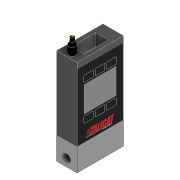
# Autodesk Inventor part: alicat_presion
Saved by Autodesk Inventor 2022 (Build 260153000, 153)
## iProperties
Created: 2022-11-14
Part Number: alicat_presion
Material: Generic
Document SubType Name: Modeling
Designer: ferna
Density: 1 g/cm^3
Appearance: Default
Author: ferna
Autodesk Inventor part; units mm, degrees
ref_plane "YZ Plane" through (0, 0, 0) normal (1, 0, 0) x (0, 1, 0)
ref_plane "XZ Plane" through (0, 0, 0) normal (0, 1, 0) x (-1, 0, 0)
ref_plane "XY Plane" through (0, 0, 0) normal (0, 0, 1) x (1, 0, 0)
sketch "Sketch1" plane through (0, 0, 0) normal (0, 1, 0) x (-1, 0, 0)
  line L0 (0, 0) -> (27, 0)
  line L1 (27, 0) -> (27, -61)
  line L2 (27, -61) -> (0, -61)
  line L3 (0, -61) -> (0, 0)
  dimension "d0" = 27
  dimension "d1" = 61
  constraints: 8 end point, 2 parallel, 1 horizontal, 1 perpendicular
  measures "d0" distance of L1.end L2.end
  measures "d1" distance of L0.end L1.end
extrude "Extrusion1" add sketch "Sketch1" along normal blind 125
sketch "Sketch2" plane through (0, 0, 0) normal (1, 0, 0) x (0, 0, -1)
  line L0 (61, 0) -> (0, 0) projected
  line L1 (61, 0) -> (61, 125) projected
  line L2 (0, 0) -> (61, 0)
  line L3 (61, 0) -> (61, 30)
  line L4 (61, 30) -> (0, 30)
  line L5 (0, 30) -> (0, 0)
  dimension "d4" = 30
  constraints: 8 end point, 2 parallel, 1 horizontal, 1 perpendicular, 1 point on line
  measures "d4" distance of L3.end L2.end
split body "Split1" sketch "Sketch2" result two bodies curves L4 L5 L2 L3 first body at (-0.5, 10, -20.3333)
sketch "Sketch3" plane through (0, 0, 0) normal (0, -1, 0) x (1, 0, 0)
  line L0 (-27, 0) -> (0, 0) projected
  line L1 (-27, -61) -> (-27, 0) projected
  line L2 (0, 0) -> (-27, -61)
  line L3 (-27, -61) -> (-22.9525, -51.8557)
  line L4 (0, 0) -> (-4.0475, -9.1443)
  circle A0 centre (-4.0475, -9.1443) radius 2
  circle A1 centre (-22.9525, -51.8557) radius 2
  line L5 (0, -61) -> (-27, -61) projected
  line L6 (-27, 0) -> (0, -61)
  line L7 (0, -61) -> (-3.238, -53.6846)
  line L8 (-27, 0) -> (-23.762, -7.3154)
  circle A2 centre (-23.762, -7.3154) radius 2
  circle A3 centre (-3.238, -53.6846) radius 2
  dimension "d5" = 10
  dimension "d6" = 10
  dimension "d7" = 4
  dimension "d8" = 4
  dimension "d14" = 8
  dimension "d15" = 8
  dimension "d16" = 4
  constraints: 12 end point, 4 centre point, 4 coincident, 4 point on line
  measures "d5" distance of L1.start L3.end
  measures "d6" distance of L0.end L4.end
  measures "d7" diameter of A0
  measures "d8" diameter of A1
  measures "d14" distance of L5.start L7.end
  measures "d15" distance of L0.start L8.end
  measures "d16" diameter of A3
extrude "Extrusion2" cut sketch "Sketch3" against normal blind 10 contours A2 L6 | L6 A2 | A3 L6 | L6 A3 bodies 2
sketch "Sketch4" plane through (-27, 0, 0) normal (0, 0, 1) x (1, 0, 0)
  line L0 (0, 0) -> (0, 30) projected
  line L1 (0, 0) -> (13.5, 0)
  line L2 (0, 0) -> (27, 0) projected
  line L3 (13.5, 0) -> (13.5, 10)
  circle A0 centre (13.5, 10) radius 5
  dimension "d11" = 10
  constraints: 4 end point, 1 centre point, 1 coincident, 1 midpoint, 1 perpendicular
  measures "d11" distance of L1.end L3.end
extrude "Extrusion3" cut sketch "Sketch4" against normal blind 10 bodies 2
sketch "Sketch12" plane through (0, 125, 0) normal (1, 0, 0) x (0, 0, -1)
  line L0 (0.5745, -8.0578) -> (59.8412, -8.0578) construction
  line L1 (59.8412, -8.0578) -> (59.8412, -95.0528) construction
  line L2 (59.8412, -95.0528) -> (0.5745, -95.0528) construction
  line L3 (0.5745, -95.0528) -> (0.5745, -8.0578) construction
  point P0 (0, -125)
  constraints: 2 other
decal "Decal2"
sketch "Sketch13" plane through (0, 125, 0) normal (0, 1, 0) x (1, 0, 0)
  line L0 (-27, 0) -> (0, 0) projected
  line L1 (0, 0) -> (-13.5, 0)
  line L2 (-13.5, 0) -> (-13.5, 30.5)
  line L3 (0, 61) -> (-27, 61) projected
  line L4 (-21.825, 46.4) -> (-5.175, 46.4)
  line L5 (-5.175, 46.4) -> (-5.175, 14.6)
  line L6 (-5.175, 14.6) -> (-21.825, 14.6)
  line L7 (-21.825, 14.6) -> (-21.825, 46.4)
  line L8 (-21.825, 46.4) -> (-5.175, 14.6) construction
  line L9 (-5.175, 46.4) -> (-21.825, 14.6) construction
  dimension "d39" = 30.5
  dimension "d40" = 16.65
  dimension "d41" = 31.8
  constraints: 16 end point, 3 midpoint, 2 parallel, 2 perpendicular, 1 horizontal
  measures "d39" distance of L1.end L2.end
  measures "d40" distance of L5.end L6.end
  measures "d41" distance of L4.end L5.end
extrude "Extrusion4" cut sketch "Sketch13" against normal blind 16.2 bodies 3
sketch "Sketch14" plane through (0, 125, 0) normal (0, 1, 0) x (1, 0, 0)
  line L0 (-5.175, 14.6) -> (-21.825, 14.6) projected
  line L1 (-13.5, 14.6) -> (-13.5, 7.3)
  line L2 (-27, 0) -> (0, 0) projected
  circle A0 centre (-13.5, 7.3) radius 4
  dimension "d44" = 7.3
  dimension "d45" = 8
  constraints: 2 end point, 1 centre point, 1 coincident, 1 midpoint, 1 perpendicular
  measures "d44" distance of L1.start L1.end
  measures "d45" diameter of A0
extrude "Extrusion5" cut sketch "Sketch14" against normal blind 1 bodies 3
sketch "Sketch15" plane through (-13.5, 124, -7.3) normal (0, 1, 0) x (1, 0, 0)
  circle A0 centre (0, 0) radius 3
  point P0 (13.5, -7.3)
  dimension "d48" = 6
  constraints: 1 centre point
  measures "d48" diameter of A0
extrude "Extrusion6" cut sketch "Sketch15" against normal blind 7 bodies 3
sketch "Sketch16" plane through (0, 125, 0) normal (0, 1, 0) x (1, 0, 0)
  circle A0 centre (-13.5, 7.3) radius 4 projected
  circle A1 centre (-13.5, 7.3) radius 3 projected
  circle A2 centre (-13.5, 7.3) radius 4.5
  point P0 (0, 0)
  dimension "d51" = 9
  constraints: 1 centre point, 1 coincident
  measures "d51" diameter of A2
extrude "Extrusion7" add sketch "Sketch16" along normal blind 10 separate body contours A0 | A1 | A2
ref_plane "Work Plane4" through (-13.5, 139, -7.3) normal (0, 1, 0) x (1, 0, 0)
sketch "Sketch17" plane through (-13.5, 139, -7.3) normal (0, 1, 0) x (1, 0, 0)
  circle A0 centre (0, 0) radius 2.5
  point P0 (13.5, -7.3)
  dimension "d55" = 5
  constraints: 1 centre point
  measures "d55" diameter of A0
extrude "Extrusion8" add sketch "Sketch17" along normal blind 5 separate body
loft "Loft1" add bodies 4 section 1 edges at (-18, 135, -7.3) section 2 edges at (-16, 139, -7.3)
combine bodies "Combine1" operation type add bodies to combine 4 5
sketch "Sketch18" plane through (-13.5, 144, -7.3) normal (0, 1, 0) x (1, 0, 0)
  circle A0 centre (0, 0) radius 2.5 projected
body "Solid4"
body "Solid2"
body "Solid3"
